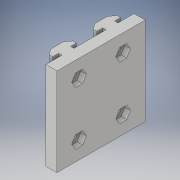
# Autodesk Inventor part: slotmountingPlate_dual_m3
Saved by Autodesk Inventor 2018 (Build 220112000, 112)
## iProperties
Created: 2020-03-14
Part Number: slotmountingPlate_dual_m3
Material: Generic
Document SubType Name: Modeling
Designer: natha
Density: 1 g/cm^3
Appearance: Default
Author: natha
Autodesk Inventor part; units mm, degrees
ref_plane "YZ Plane" through (0, 0, 0) normal (1, 0, 0) x (0, 1, 0)
ref_plane "XZ Plane" through (0, 0, 0) normal (0, 1, 0) x (-1, 0, 0)
ref_plane "XY Plane" through (0, 0, 0) normal (0, 0, 1) x (1, 0, 0)
sketch "Sketch1" plane through (0, 0, 0) normal (0, 1, 0) x (-1, 0, 0)
  line L0 (0, -5.4) -> (1.5, -5.4)
  line L1 (1.5, -5.4) -> (1.5, -8.1)
  line L2 (1.5, -8.1) -> (3.2, -8.1)
  line L3 (0, 0) -> (1.5, 0)
  line L4 (1.5, 0) -> (1.5, 2.7)
  line L5 (1.5, 2.7) -> (3.2, 2.7)
  line L6 (5, 0) -> (5, -5.4)
  line L7 (5, -5.4) -> (3.2, -8.1)
  line L8 (5, 0) -> (3.2, 2.7)
  line L9 (0, -20) -> (1.5, -20)
  line L10 (1.5, -20) -> (1.5, -17.3)
  line L11 (1.5, -17.3) -> (3.2, -17.3)
  line L12 (0, -25.4) -> (1.5, -25.4)
  line L13 (1.5, -25.4) -> (1.5, -28.1)
  line L14 (1.5, -28.1) -> (3.2, -28.1)
  line L15 (5, -20) -> (5, -25.4)
  line L16 (5, -25.4) -> (3.2, -28.1)
  line L17 (5, -20) -> (3.2, -17.3)
  line L18 (0, -5.4) -> (0, -20)
  line L19 (0, 0) -> (0, 7.3)
  line L20 (0, 7.3) -> (-5, 7.3)
  line L21 (0, -25.4) -> (0, -32.7)
  line L22 (0, -32.7) -> (-5, -32.7)
  line L23 (-5, -32.7) -> (-5, 7.3)
  dimension "d0" = 5.4
  dimension "d1" = 1.5
  dimension "d2" = 2.7
  dimension "d3" = 1.7
  dimension "d4" = 2.7
  dimension "d5" = 1.7
  dimension "d9" = 2.7
  dimension "d10" = 2.7
  dimension "d11" = 5.4
  dimension "d12" = 7.3
  dimension "d13" = 5
  dimension "d14" = 7.3
  dimension "d15" = 5
  dimension "d16" = 20
  constraints: 48 end point, 11 perpendicular, 4 vertical, 3 horizontal, 1 parallel
  measures "d0" distance of L3.start L0.start
  measures "d1" distance of L0.start L0.end
  measures "d2" distance of L0.end L1.end
  measures "d3" distance of L1.end L2.end
  measures "d4" distance of L3.end L4.end
  measures "d5" distance of L4.end L5.end
  measures "d9" distance of L9.end L10.end
  measures "d10" distance of L12.end L13.end
  measures "d11" distance between parallel lines of L12 L9
  measures "d12" distance of L3.start L19.end
  measures "d13" distance of L19.end L20.end
  measures "d14" distance of L12.start L21.end
  measures "d15" distance of L21.end L22.end
  measures "d16" distance between parallel lines of L3 L9
extrude "Extrusion1" add sketch "Sketch1" along normal blind 40
sketch "Sketch2" plane through (5, 0, 7.3) normal (1, 0, 0) x (0, 0, -1)
  line L0 (11.6599, 5) -> (8.3401, 5)
  line L1 (8.3401, 5) -> (6.6802, 7.875)
  line L2 (6.6802, 7.875) -> (8.3401, 10.75)
  line L3 (8.3401, 10.75) -> (11.6599, 10.75)
  line L4 (11.6599, 10.75) -> (13.3198, 7.875)
  line L5 (13.3198, 7.875) -> (11.6599, 5)
  line L6 (40, 0) -> (0, 0) projected
  line L7 (0, 0) -> (0, 40) projected
  line L8 (31.6599, 5) -> (28.3401, 5)
  line L9 (28.3401, 5) -> (26.6802, 7.875)
  line L10 (26.6802, 7.875) -> (28.3401, 10.75)
  line L11 (28.3401, 10.75) -> (31.6599, 10.75)
  line L12 (31.6599, 10.75) -> (33.3198, 7.875)
  line L13 (33.3198, 7.875) -> (31.6599, 5)
  line L14 (40, 0) -> (40, 40) projected
  line L15 (11.6599, 29.25) -> (8.3401, 29.25)
  line L16 (8.3401, 29.25) -> (6.6802, 32.125)
  line L17 (6.6802, 32.125) -> (8.3401, 35)
  line L18 (8.3401, 35) -> (11.6599, 35)
  line L19 (11.6599, 35) -> (13.3198, 32.125)
  line L20 (13.3198, 32.125) -> (11.6599, 29.25)
  line L21 (31.6599, 29.25) -> (28.3401, 29.25)
  line L22 (28.3401, 29.25) -> (26.6802, 32.125)
  line L23 (26.6802, 32.125) -> (28.3401, 35)
  line L24 (28.3401, 35) -> (31.6599, 35)
  line L25 (31.6599, 35) -> (33.3198, 32.125)
  line L26 (33.3198, 32.125) -> (31.6599, 29.25)
  line L27 (0, 40) -> (40, 40) projected
  point P0 (7.3, 0)
  point P1 (10, 7.875)
  point P2 (30, 7.875)
  point P3 (10, 32.125)
  point P4 (30, 32.125)
  dimension "d17" = 5.75
  dimension "d18" = 5
  dimension "d19" = 10
  dimension "d20" = 5.75
  dimension "d21" = 5
  dimension "d22" = 10
  dimension "d23" = 5.75
  dimension "d24" = 5.75
  dimension "d25" = 5
  dimension "d26" = 5
  dimension "d27" = 10
  dimension "d28" = 10
  constraints: 48 end point, 4 parallel, 52 other
  measures "d17" distance between parallel lines of L3 L0
  measures "d18" distance between parallel lines of L6 L0
  measures "d19" distance from line of L7 point (10, 7.875)
  measures "d20" distance between parallel lines of L11 L8
  measures "d21" distance between parallel lines of L6 L8
  measures "d22" distance from line of L14 point (30, 7.875)
  measures "d23" distance between parallel lines of L15 L18
  measures "d24" distance between parallel lines of L21 L24
  measures "d25" distance between parallel lines of L18 L27
  measures "d26" distance between parallel lines of L27 L24
  measures "d27" distance from line of L7 point (10, 32.125)
  measures "d28" distance from line of L14 point (30, 32.125)
extrude "Extrusion2" cut sketch "Sketch2" against normal blind 2.5 contours L0 L1 L2 L3 L4 L5 | L8 L9 L10 L11 L12 L13 | L15 L16 L17 L18 L19 L20 | L21 L22 L23 L24 L25 L26
sketch "Sketch3" plane through (2.5, 0, 7.3) normal (1, 0, 0) x (0, 0, -1)
  circle A0 centre (30, 7.75) radius 1.375
  circle A1 centre (10, 7.75) radius 1.375
  circle A2 centre (10, 32.25) radius 1.375
  circle A3 centre (30, 32.25) radius 1.375
  point P0 (7.3, 0)
  dimension "d31" = 2.75
  dimension "d32" = 2.75
  dimension "d33" = 2.75
  constraints: 4 centre point
  measures "d31" diameter of A0
  measures "d32" diameter of A1
  measures "d33" diameter of A2
extrude "Extrusion3" cut sketch "Sketch3" against normal blind 20
body "Solid1"
